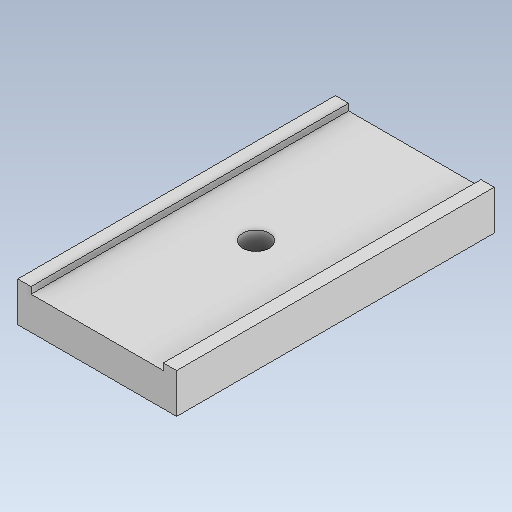
# Autodesk Inventor part: centershortNEW
Saved by Autodesk Inventor 2020 (Build 240168000, 168)
## iProperties
Created: 2019-12-18
Part Number: centershortNEW
Material: Generic
Document SubType Name: Modeling
Designer: xj82b
Density: 1 g/cm^3
Appearance: Default
Author: xj82b
Autodesk Inventor part; units mm, degrees
ref_plane "YZ Plane" through (0, 0, 0) normal (1, 0, 0) x (0, 1, 0)
ref_plane "XZ Plane" through (0, 0, 0) normal (0, 1, 0) x (-1, 0, 0)
ref_plane "XY Plane" through (0, 0, 0) normal (0, 0, 1) x (1, 0, 0)
sketch "Sketch1" plane through (0, 0, 0) normal (0, 1, 0) x (-1, 0, 0)
  line L0 (0, 0) -> (-24, 0)
  line L1 (-24, 0) -> (-24, -48)
  line L2 (-24, -48) -> (0, -48)
  line L3 (0, -48) -> (0, 0)
  circle A0 centre (-12, -24) radius 2
  point P0 (-24, -24)
  point P1 (-12, 0)
  dimension "d0" = 24
  dimension "d1" = 48
  dimension "d2" = 4
  constraints: 8 end point, 2 midpoint, 2 parallel, 1 centre point, 1 horizontal, 1 horizontal alignment, 1 perpendicular, 1 vertical alignment
  measures "d0" distance of L2.end L1.end
  measures "d1" distance of L1.end L0.end
  measures "d2" diameter of A0
extrude "Extrusion1" add sketch "Sketch1" along normal blind 6
sketch "Sketch2" plane through (0, 6, 0) normal (0, 1, 0) x (1, 0, 0)
  line L0 (2, 75.3172) -> (22, 75.3172)
  line L1 (22, 75.3172) -> (22, -3.0502)
  line L2 (22, -3.0502) -> (2, -3.0502)
  line L3 (2, -3.0502) -> (2, 75.3172)
  line L4 (0, 48) -> (0, 0) projected
  dimension "d5" = 20
  dimension "d6" = 2
  constraints: 8 end point, 2 parallel, 1 horizontal, 1 perpendicular
  measures "d5" distance of L0.start L0.end
  measures "d6" distance between parallel lines of L4 L3
extrude "Extrusion2" cut sketch "Sketch2" against normal blind 1
body "Solid1"
